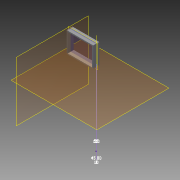
# Autodesk Inventor part: central_foot
Saved by Autodesk Inventor 2015 SP1 (Build 190203100, 203)
## iProperties
Created: 2016-03-25
Part Number: central_foot
Material: Generic
Document SubType Name: Modeling
Designer: Alexandre Cherpillod
Density: 1 g/cm^3
Appearance: Default
Mass: 3.01 g
Surface Area: 36.12 cm^2
Volume: 3.01 cm^3
Author: Alexandre Cherpillod
Autodesk Inventor part; units mm, degrees
ref_plane "XZ Plane" through (0, 0, 0) normal (0, 1, 0) x (-1, 0, 0)
sketch "Sketch1" plane through (0, 0, 0) normal (0, 1, 0) x (-1, 0, 0)
  line L0 (0, 0) -> (-40.5, 0)
  line L1 (-40.5, 0) -> (-40.5, 30.75)
  line L2 (-40.5, 30.75) -> (0, 30.75)
  line L3 (0, 30.75) -> (0, 0)
  line L4 (2, 32.75) -> (-42.5, 32.75)
  line L5 (-42.5, 32.75) -> (-42.5, -2)
  line L6 (-42.5, -2) -> (2, -2)
  line L7 (2, -2) -> (2, 32.75)
  dimension "d2" = 40.5
  dimension "d3" = 30.75
  dimension "d4" = 2
  constraints: 16 end point, 4 parallel, 2 perpendicular, 1 horizontal, 3 other
  measures "d2" distance of L1.end L2.end
  measures "d3" distance of L0.end L1.end
  measures "d4" distance between parallel lines of L2 L4
extrude "Extrusion1" add sketch "Sketch1" along normal blind 10
ref_plane "Work Plane19" through (0, 5, 0) normal (0, 1, 0) x (1, 0, 0)
ref_plane "Work Plane20" through (42.5, 5, 32.75) normal (-0.7071, -0.7071, 0) x (0, 0, 1)
sketch "Sketch2" plane through (42.5, 5, 32.75) normal (-0.7071, -0.7071, 0) x (0, 0, 1)
  line L0 (0, -3.5355) -> (-34.75, -3.5355) construction
  line L1 (-34.75, -3.5355) -> (-34.75, 3.5355) construction
  line L2 (0, 3.5355) -> (-34.75, 3.5355) construction
  line L3 (0, -3.5355) -> (0, 3.5355) construction
  line L4 (-41.7, 0) -> (6.95, 0) construction
  line L5 (-34.75, 0) -> (-86.722, -105.5837)
  line L6 (-32.75, 33.5876) -> (-32.75, 4.9497) projected
  arc A0 (-86.722, -105.5837) -> (-80.0972, -119.7206) centre (-77.75, -110) ccw construction
  line L7 (-87.75, -113.6702) -> (-87.75, -110) construction
  line L8 (-87.75, -110) -> (-87.75, -104.3872) construction
  arc A1 (-86.722, -105.5837) -> (-87.75, -110) centre (-77.75, -110) ccw
  arc A2 (-87.75, -110) -> (-84.8211, -117.0711) centre (-77.75, -110) ccw
  point P0 (-32.75, 26.5165)
  dimension "d15" = 110
  dimension "d16" = 55
  dimension "d21" = 45
  dimension "d22" = 10
  constraints: 7 point on circle, 6 end point, 3 centre point, 3 tangent, 2 coincident, 2 vertical, 1 midpoint, 1 point on line
  measures "d15" distance from line of L4 L7.end
  measures "d16" distance from line of L6 L7.end
  measures "d22" radius of A0
body "Solid1"
